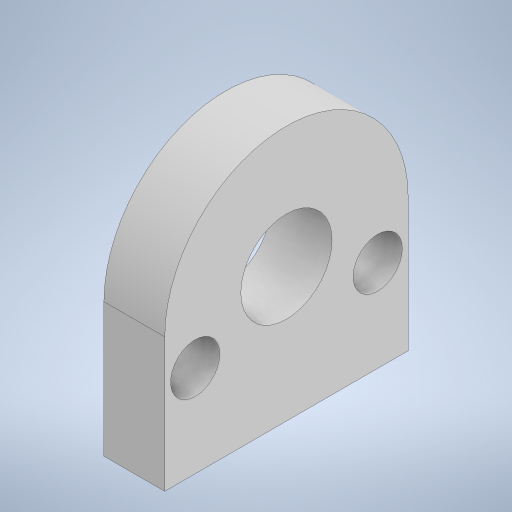
# Autodesk Inventor part: arco_obj4
Saved by Autodesk Inventor 2023.2 (Build 272271030, 271C)
## iProperties
Created: 2023-02-25
Part Number: arco_obj4
Material: Generic
Document SubType Name: Modeling
Designer: Cris Pat
Density: 1 g/cm^3
Appearance: Default
Author: Cris Pat
Autodesk Inventor part; units mm, degrees
ref_plane "YZ Plane" through (0, 0, 0) normal (1, 0, 0) x (0, 1, 0)
ref_plane "XZ Plane" through (0, 0, 0) normal (0, 1, 0) x (-1, 0, 0)
ref_plane "XY Plane" through (0, 0, 0) normal (0, 0, 1) x (1, 0, 0)
sketch "Sketch1" plane through (0, 0, 0) normal (1, 0, 0) x (0, 1, 0)
  line L0 (-11, -20) -> (11, -20)
  arc A0 (11, -20) -> (11, 20) centre (11, 0) ccw
  line L1 (11, 20) -> (-11, 20)
  line L2 (-11, 20) -> (-11, -20)
  circle A1 centre (11, 0) radius 7.5
  point P0 (0, 0)
  point P1 (0, -20)
  dimension "d0" = 22
  dimension "d1" = 22
  dimension "d2" = 40
  dimension "d3" = 15
  constraints: 6 end point, 2 centre point, 2 point on circle, 2 tangent, 1 coincident, 1 horizontal, 1 horizontal alignment, 1 midpoint, 1 parallel, 1 vertical alignment
  measures "d0" distance of L0.start L0.end
  measures "d1" distance of L1.start L1.end
  measures "d2" distance of L1.end L0.start
  measures "d3" diameter of A1
extrude "Extrusion1" add sketch "Sketch1" along normal mid plane 10
sketch "Sketch2" plane through (5, 0, 0) normal (1, 0, 0) x (0, 0, -1)
  arc A0 (20, 11) -> (-20, 11) centre (0, 11) ccw construction
  line L0 (-20, 11) -> (-20, -11) construction
  line L1 (-20, -11) -> (20, -11) construction
  line L2 (20, -11) -> (20, 11) construction
  circle A1 centre (0, 11) radius 7.5 construction
  circle A2 centre (15, 4.05) radius 4.05
  line L3 (0, 11) -> (0, -11) construction
  line L4 (-20, -11) -> (20, -11) construction
  circle A3 centre (-15, 4.05) radius 4.05
  point P0 (0, 0)
  dimension "d6" = 15.05
  dimension "d7" = 8.1
  dimension "d8" = 5
  constraints: 2 centre point, 2 end point, 1 midpoint, 1 symmetric about line, 1 other
  measures "d6" distance from line of L1 A2.centre
  measures "d7" diameter of A2
  measures "d8" distance from line of L2 A2.centre
extrude "Extrusion2" cut sketch "Sketch2" against normal through all
body "Solid1"
